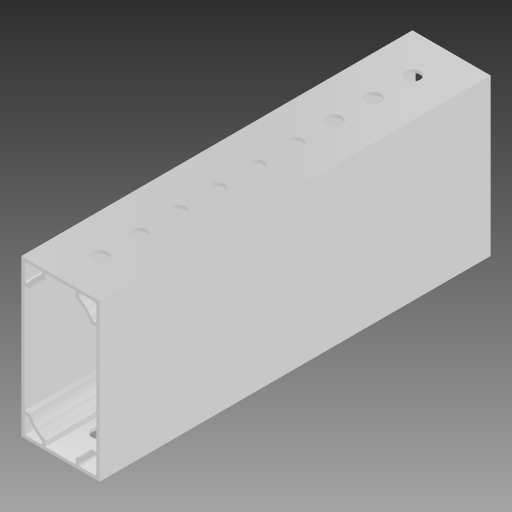
# Autodesk Inventor part: REVLIFT-MAXTubes
Saved by Autodesk Inventor 2023 (Build 270158000, 158)
## iProperties
Created: 2022-12-30
Part Number: REVLIFT-MAXTubes
Material: Aluminum 6061
Document SubType Name: Modeling
Designer: Max Boord
Mass: 64.8858 g
Surface Area: 460.618 cm^2
Volume: 24.0318 cm^3
Density: 2.7 g/cm^3
Appearance: Aluminum - Dark
Mass: 511.861 g
Surface Area: 3609.21 cm^2
Volume: 189.578 cm^3
Author: Max Boord
Mass: 63.7381 g
Surface Area: 454.736 cm^2
Volume: 23.6067 cm^3
Mass: 155.576 g
Surface Area: 1099.46 cm^2
Volume: 57.6209 cm^3
Autodesk Inventor part; units mm, degrees
ref_plane "YZ Plane" through (0, 0, 0) normal (1, 0, 0) x (0, 1, 0)
ref_plane "XZ Plane" through (0, 0, 0) normal (0, 1, 0) x (-1, 0, 0)
ref_plane "XY Plane" through (0, 0, 0) normal (0, 0, 1) x (1, 0, 0)
sketch "Thin Wall 2x1 MAXTube" plane through (0, 0, 0) normal (0, 0, 1) x (1, 0, 0)
  line L0 (1.016, 42.9895) -> (1.016, 7.8105)
  line L1 (2.721, 42.9895) -> (1.016, 42.9895)
  arc A0 (7.8105, 48.079) -> (2.721, 42.9895) centre (12.7, 38.1) ccw
  line L2 (7.8105, 49.784) -> (7.8105, 48.079)
  line L3 (17.5895, 49.784) -> (7.8105, 49.784)
  line L4 (17.5895, 48.079) -> (17.5895, 49.784)
  arc A1 (22.679, 42.9895) -> (17.5895, 48.079) centre (12.7, 38.1) ccw
  line L5 (24.384, 42.9895) -> (22.679, 42.9895)
  line L6 (24.384, 7.8105) -> (24.384, 42.9895)
  line L7 (22.679, 7.8105) -> (24.384, 7.8105)
  arc A2 (17.5895, 2.721) -> (22.679, 7.8105) centre (12.7, 12.7) ccw
  line L8 (17.5895, 1.016) -> (17.5895, 2.721)
  line L9 (7.8105, 1.016) -> (17.5895, 1.016)
  line L10 (7.8105, 2.721) -> (7.8105, 1.016)
  arc A3 (2.721, 7.8105) -> (7.8105, 2.721) centre (12.7, 12.7) ccw
  line L11 (1.016, 7.8105) -> (2.721, 7.8105)
  arc A4 (6.4588, 48.4994) -> (6.1029, 49.784) centre (6.1029, 49.0924) ccw
  arc A5 (6.4588, 48.4994) -> (2.3006, 44.3412) centre (12.7, 38.1) ccw
  arc A6 (1.016, 44.6971) -> (2.3006, 44.3412) centre (1.7076, 44.6971) ccw
  line L12 (1.016, 49.0924) -> (1.016, 44.6971)
  arc A7 (1.7076, 49.784) -> (1.016, 49.0924) centre (1.7076, 49.0924) ccw
  line L13 (6.1029, 49.784) -> (1.7076, 49.784)
  arc A8 (18.9412, 2.3006) -> (19.2971, 1.016) centre (19.2971, 1.7076) ccw
  arc A9 (18.9412, 2.3006) -> (23.0994, 6.4588) centre (12.7, 12.7) ccw
  arc A10 (24.384, 6.1029) -> (23.0994, 6.4588) centre (23.6924, 6.1029) ccw
  line L14 (24.384, 1.7076) -> (24.384, 6.1029)
  arc A11 (23.6924, 1.016) -> (24.384, 1.7076) centre (23.6924, 1.7076) ccw
  line L15 (19.2971, 1.016) -> (23.6924, 1.016)
  arc A12 (24.384, 49.0924) -> (23.6924, 49.784) centre (23.6924, 49.0924) ccw
  line L16 (24.384, 44.6971) -> (24.384, 49.0924)
  arc A13 (23.0994, 44.3412) -> (24.384, 44.6971) centre (23.6924, 44.6971) ccw
  arc A14 (23.0994, 44.3412) -> (18.9412, 48.4994) centre (12.7, 38.1) ccw
  arc A15 (19.2971, 49.784) -> (18.9412, 48.4994) centre (19.2971, 49.0924) ccw
  line L17 (23.6924, 49.784) -> (19.2971, 49.784)
  line L18 (25.4, 0) -> (0, 0)
  line L19 (25.4, 50.8) -> (25.4, 0)
  line L20 (0, 50.8) -> (25.4, 50.8)
  line L21 (0, 0) -> (0, 50.8)
  arc A16 (1.016, 1.7076) -> (1.7076, 1.016) centre (1.7076, 1.7076) ccw
  line L22 (1.016, 6.1029) -> (1.016, 1.7076)
  arc A17 (2.3006, 6.4588) -> (1.016, 6.1029) centre (1.7076, 6.1029) ccw
  arc A18 (2.3006, 6.4588) -> (6.4588, 2.3006) centre (12.7, 12.7) ccw
  arc A19 (6.1029, 1.016) -> (6.4588, 2.3006) centre (6.1029, 1.7076) ccw
  line L23 (1.7076, 1.016) -> (6.1029, 1.016)
  point P0 (12.7, 25.4)
  point P1 (12.7, 25.4)
  point P2 (12.7, 49.784)
  point P3 (12.7, 50.8)
  point P4 (12.7, 1.016)
  point P5 (12.7, 0)
  point P6 (0, 25.4)
  point P7 (1.016, 25.4)
  point P8 (24.384, 25.4)
  point P9 (25.4, 25.4)
  dimension "d0" = 25.4
  dimension "d1" = 50.8
  dimension "d2" = 1.016
  dimension "d3" = 1.016
  dimension "d4" = 12.7
  dimension "d5" = 12.7
  dimension "d6" = 9.779
  dimension "d7" = 35.179
  measures "d0" distance between parallel lines of L19 L21
  measures "d1" distance between parallel lines of L18 L20
  measures "d2" distance between parallel lines of L0 L21
  measures "d3" distance between parallel lines of L3 L20
  measures "d4" distance of point (12.7, 25.4) A0.centre
  measures "d5" distance of point (12.7, 25.4) A2.centre
  measures "d6" distance between parallel lines of L4 L2
  measures "d7" distance between parallel lines of L11 L1
sketch "Sketch1" plane through (0, 0, 0) normal (0, 0, 1) x (1, 0, 0)
  line L0 (-11.684, 17.5895) -> (-11.684, -17.5895)
  line L1 (-9.979, 17.5895) -> (-11.684, 17.5895)
  arc A0 (-4.8895, 22.679) -> (-9.979, 17.5895) centre (0, 12.7) ccw
  line L2 (-4.8895, 24.384) -> (-4.8895, 22.679)
  line L3 (4.8895, 24.384) -> (-4.8895, 24.384)
  line L4 (4.8895, 22.679) -> (4.8895, 24.384)
  arc A1 (9.979, 17.5895) -> (4.8895, 22.679) centre (0, 12.7) ccw
  line L5 (11.684, 17.5895) -> (9.979, 17.5895)
  line L6 (11.684, -17.5895) -> (11.684, 17.5895)
  line L7 (9.979, -17.5895) -> (11.684, -17.5895)
  arc A2 (4.8895, -22.679) -> (9.979, -17.5895) centre (0, -12.7) ccw
  line L8 (4.8895, -24.384) -> (4.8895, -22.679)
  line L9 (-4.8895, -24.384) -> (4.8895, -24.384)
  line L10 (-4.8895, -22.679) -> (-4.8895, -24.384)
  arc A3 (-9.979, -17.5895) -> (-4.8895, -22.679) centre (0, -12.7) ccw
  line L11 (-11.684, -17.5895) -> (-9.979, -17.5895)
  arc A4 (-6.2412, 23.0994) -> (-6.5971, 24.384) centre (-6.5971, 23.6924) ccw
  arc A5 (-6.2412, 23.0994) -> (-10.3994, 18.9412) centre (0, 12.7) ccw
  arc A6 (-11.684, 19.2971) -> (-10.3994, 18.9412) centre (-10.9924, 19.2971) ccw
  line L12 (-11.684, 23.6924) -> (-11.684, 19.2971)
  arc A7 (-10.9924, 24.384) -> (-11.684, 23.6924) centre (-10.9924, 23.6924) ccw
  line L13 (-6.5971, 24.384) -> (-10.9924, 24.384)
  arc A8 (6.2412, -23.0994) -> (6.5971, -24.384) centre (6.5971, -23.6924) ccw
  arc A9 (6.2412, -23.0994) -> (10.3994, -18.9412) centre (0, -12.7) ccw
  arc A10 (11.684, -19.2971) -> (10.3994, -18.9412) centre (10.9924, -19.2971) ccw
  line L14 (11.684, -23.6924) -> (11.684, -19.2971)
  arc A11 (10.9924, -24.384) -> (11.684, -23.6924) centre (10.9924, -23.6924) ccw
  line L15 (6.5971, -24.384) -> (10.9924, -24.384)
  arc A12 (11.684, 23.6924) -> (10.9924, 24.384) centre (10.9924, 23.6924) ccw
  line L16 (11.684, 19.2971) -> (11.684, 23.6924)
  arc A13 (10.3994, 18.9412) -> (11.684, 19.2971) centre (10.9924, 19.2971) ccw
  arc A14 (10.3994, 18.9412) -> (6.2412, 23.0994) centre (0, 12.7) ccw
  arc A15 (6.5971, 24.384) -> (6.2412, 23.0994) centre (6.5971, 23.6924) ccw
  line L17 (10.9924, 24.384) -> (6.5971, 24.384)
  line L18 (12.7, -25.4) -> (-12.7, -25.4)
  line L19 (12.7, 25.4) -> (12.7, -25.4)
  line L20 (-12.7, 25.4) -> (12.7, 25.4)
  line L21 (-12.7, -25.4) -> (-12.7, 25.4)
  arc A16 (-11.684, -23.6924) -> (-10.9924, -24.384) centre (-10.9924, -23.6924) ccw
  line L22 (-11.684, -19.2971) -> (-11.684, -23.6924)
  arc A17 (-10.3994, -18.9412) -> (-11.684, -19.2971) centre (-10.9924, -19.2971) ccw
  arc A18 (-10.3994, -18.9412) -> (-6.2412, -23.0994) centre (0, -12.7) ccw
  arc A19 (-6.5971, -24.384) -> (-6.2412, -23.0994) centre (-6.5971, -23.6924) ccw
  line L23 (-10.9924, -24.384) -> (-6.5971, -24.384)
  point P0 (0, 0)
  constraints: 1 other
extrude "Extrusion1" add sketch "Sketch1" along normal mid plane 127
sketch "Sketch2" plane through (-12.7, -25.4, 63.5) normal (-1, 0, 0) x (0, 0, 1)
  line L0 (0, 50.8) -> (-127, 50.8) projected
  line L1 (0, 0) -> (0, 50.8) projected
  line L2 (-127, 0) -> (0, 0) projected
  line L3 (-127, 50.8) -> (-127, 0) projected
  line L4 (0, 50.8) -> (-127, 0)
  point P0 (-63.5, 25.4)
  constraints: 2 end point
hole "Hole1" [suppressed]
pattern_linear "Rectangular Pattern1" [suppressed]
sketch "Sketch3" plane through (-12.7, 25.4, 63.5) normal (0, 1, 0) x (1, 0, 0)
  point P0 (12.7, 63.5)
hole "Hole2" at (0, 25.4, 0) direction (0, -1, 0) diameter 4.9784 end through all
pattern_linear "Rectangular Pattern2" count 9 spacing 12.7 along (0, 0, 1) of "Hole2" first direction both ways yes
sketch "Sketch5" plane through (12.7, -25.4, 63.5) normal (1, 0, 0) x (0, 0, -1)
  line L0 (0, 50.8) -> (127, 50.8) projected
  line L1 (0, 0) -> (0, 50.8) projected
  line L2 (127, 0) -> (0, 0) projected
  line L3 (127, 50.8) -> (127, 0) projected
  circle A0 centre (11.3538, 38.1) radius 2.4892
  circle A1 centre (24.0538, 38.1) radius 2.4892
  circle A2 centre (36.7538, 38.1) radius 2.4892
  circle A3 centre (11.3538, 12.7) radius 2.4892
  circle A4 centre (24.0538, 12.7) radius 2.4892
  circle A5 centre (36.7538, 12.7) radius 2.4892
  line L4 (11.3538, 38.1) -> (0, 25.4) construction
  line L5 (0, 50.8) -> (0, 0) projected
  line L6 (11.3538, 12.7) -> (0, 25.4) construction
  point P0 (63.5, 25.4)
  dimension "d35" = 4.9784
  dimension "d38" = 12.7
  dimension "d41" = 25.4
  dimension "d44" = 11.3538
  constraints: 6 centre point, 4 end point, 2 midpoint, 1 equal length, 1 horizontal, 1 vertical, 10 other
  measures "d35" diameter of A0
  measures "d38" distance of L4.start A1.centre
  measures "d41" distance of L4.start L6.start
  measures "d44" horizontal distance of point (0, 25.4) L4.start
extrude "Extrusion4" [suppressed]
sketch "Sketch6" plane through (12.7, -25.4, 63.5) normal (1, 0, 0) x (0, 0, -1)
  circle A0 centre (12.7, 38.1) radius 2.4892 projected
  circle A1 centre (25.4, 38.1) radius 2.4892 projected
  circle A2 centre (38.1, 38.1) radius 2.4892 projected
  circle A3 centre (12.7, 12.7) radius 2.4892 projected
  circle A4 centre (25.4, 12.7) radius 2.4892 projected
  circle A5 centre (38.1, 12.7) radius 2.4892 projected
  point P0 (63.5, 25.4)
  point P1 (12.7, 38.1)
  point P2 (25.4, 38.1)
  point P3 (38.1, 38.1)
  point P4 (12.7, 12.7)
  point P5 (25.4, 12.7)
  point P6 (38.1, 12.7)
  constraints: 6 coincident
hole "Hole3" [suppressed]
body "Solid1"
